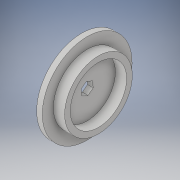
# Autodesk Inventor part: wheel hub
Saved by Autodesk Inventor 2018 (Build 220112000, 112)
## iProperties
Created: 2018-01-26
Part Number: wheel hub
Material: Generic
Document SubType Name: Modeling
Designer: prakh
Density: 1 g/cm^3
Appearance: Default
Author: prakh
Autodesk Inventor part; units mm, degrees
ref_plane "YZ Plane" through (0, 0, 0) normal (1, 0, 0) x (0, 1, 0)
ref_plane "XZ Plane" through (0, 0, 0) normal (0, 1, 0) x (-1, 0, 0)
ref_plane "XY Plane" through (0, 0, 0) normal (0, 0, 1) x (1, 0, 0)
sketch "Sketch1" plane through (0, 0, 0) normal (1, 0, 0) x (0, 1, 0)
  circle A0 centre (0, 0) radius 50.546
  dimension "d0" = 101.092
  constraints: 1 centre point, 1 coincident
  measures "d0" diameter of A0
extrude "Extrusion1" add sketch "Sketch1" along normal blind 6.35
sketch "Sketch2" plane through (6.35, 0, 0) normal (1, 0, 0) x (0, 0, -1)
  circle A0 centre (0, 0) radius 38.1
  circle A1 centre (0, 0) radius 31.75
  dimension "d3" = 76.2
  dimension "d4" = 6.35
  constraints: 2 centre point, 2 coincident
  measures "d3" diameter of A0
  measures "d4" radial gap between concentric circles of A1 A0
extrude "Extrusion2" add sketch "Sketch2" along normal blind 12.7
sketch "Sketch3" plane through (6.35, 0, 0) normal (1, 0, 0) x (0, 0, -1)
  line L0 (-6.7678, 2.8213) -> (-0.9406, 7.2718)
  line L1 (-0.9406, 7.2718) -> (5.8273, 4.4504)
  line L2 (5.8273, 4.4504) -> (6.7678, -2.8213)
  line L3 (6.7678, -2.8213) -> (0.9406, -7.2718)
  line L4 (0.9406, -7.2718) -> (-5.8273, -4.4504)
  line L5 (-5.8273, -4.4504) -> (-6.7678, 2.8213)
  point P0 (0, 0)
  point P1 (0, 0)
  dimension "d7" = 12.7
  constraints: 12 end point, 1 coincident, 13 other
  measures "d7" distance between parallel lines of L3 L0
extrude "Extrusion3" cut sketch "Sketch3" against normal blind 12.7
body "Solid1"
